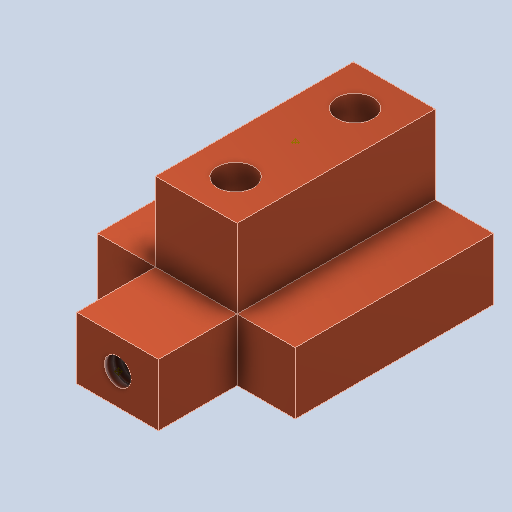
# Autodesk Inventor part: copper_top_ledgereod
Saved by Autodesk Inventor 2024.2 (Build 282272000, 272)
## iProperties
Created: 2023-03-13
Part Number: copper_top_ledgereod
Material: Copper
Document SubType Name: Modeling
Designer: warke
Density: 8.94 g/cm^3
Appearance: Copper - Satin
Author: warke
Autodesk Inventor part; units mm, degrees
ref_plane "YZ Plane" through (0, 0, 0) normal (1, 0, 0) x (0, 1, 0)
ref_plane "XZ Plane" through (0, 0, 0) normal (0, 1, 0) x (-1, 0, 0)
ref_plane "XY Plane" through (0, 0, 0) normal (0, 0, 1) x (1, 0, 0)
sketch "Sketch1" plane through (0, 0, 0) normal (0, 1, 0) x (-1, 0, 0)
  point P0 (0, 0)
sketch "Sketch2" plane through (0, 0, 0) normal (0, 1, 0) x (-1, 0, 0)
  line L0 (3.3, 8) -> (-3.3, 8)
  line L1 (-3.3, 8) -> (-3.3, -8)
  line L2 (-3.3, -8) -> (3.3, -8)
  line L3 (3.3, -8) -> (3.3, 8)
  line L4 (3.3, 8) -> (-3.3, -8) construction
  line L5 (-3.3, 8) -> (3.3, -8) construction
  point P0 (0, 0)
  dimension "d0" = 6.6
  dimension "d1" = 16
  constraints: 12 end point, 2 midpoint, 2 parallel, 1 horizontal, 1 perpendicular
  measures "d0" distance of L2.end L1.end
  measures "d1" distance of L1.end L0.end
extrude "Extrusion1" add sketch "Sketch2" along normal blind 6.35
sketch "Sketch3" plane through (0, 0, 0) normal (0, -1, 0) x (1, 0, 0)
  line L0 (-8, -8) -> (8, -8)
  line L1 (8, -8) -> (8, 8)
  line L2 (8, 8) -> (-8, 8)
  line L3 (-8, 8) -> (-8, -8)
  line L4 (-8, -8) -> (8, 8) construction
  line L5 (8, -8) -> (-8, 8) construction
  point P0 (0, 0)
  dimension "d13" = 16
  dimension "d14" = 16
  constraints: 12 end point, 2 midpoint, 2 parallel, 1 horizontal, 1 perpendicular
  measures "d13" distance of L2.end L1.end
  measures "d14" distance of L1.end L0.end
move or copy body "Move1" bodies to move or copy 1 copy no translate (0, 6.35, 0)
extrude "Extrusion2" add sketch "Sketch3" against normal up to surface (6.35 mm away)
chamfer "Chamfer1" [suppressed]
chamfer "Chamfer2" [suppressed]
sketch "Sketch4" plane through (-3.3, 12.7, -8) normal (0, 1, 0) x (1, 0, 0)
  line L0 (4.4354, -16) -> (2.1646, -16) projected
  line L1 (-4.7, 0) -> (11.3, 0) projected
  point P0 (3.3, -8)
  point P1 (3.3, -3.175)
  point P2 (3.3, -12.825)
fillet "Fillet1" [suppressed]
sketch "Sketch5" plane through (-3.3, 12.7, 8) normal (0, 0, 1) x (1, 0, 0)
  circle A0 centre (3.3, -9.5232) radius 2.9337
  point P0 (3.3, -12.7)
  constraints: 1 centre point, 1 coincident
extrude "Extrusion3" [suppressed]
hole "Hole3" [suppressed]
chamfer "Chamfer3" [suppressed]
sketch "Sketch6" plane through (-3.3, 12.7, -8) normal (-1, 0, 0) x (0, 0, 1)
  line L0 (0, 0) -> (16, 0) projected
  circle A0 centre (8, -2.27) radius 1.27
  point P0 (8, -12.7)
  dimension "d62" = 2.54
  constraints: 1 centre point
  measures "d62" diameter of A0
extrude "Extrusion4" cut sketch "Sketch6" against normal blind 3.3
sketch "Sketch7" plane through (-3.3, 12.7, 8) normal (0, 0, 1) x (1, 0, 0)
  line L0 (0, -6.35) -> (0, 0) projected
  line L1 (11.3, -12.7) -> (-4.7, -12.7) projected
  line L2 (0, -6.35) -> (6.6, -6.35)
  line L3 (6.6, -6.35) -> (6.6, -12.7)
  line L4 (6.6, -12.7) -> (0, -12.7)
  line L5 (0, -12.7) -> (0, -6.35)
  point P0 (3.3, -12.7)
  dimension "d65" = 6.6
  constraints: 8 end point, 2 parallel, 1 horizontal, 1 perpendicular, 1 point on line
  measures "d65" distance of L3.end L4.end
extrude "Extrusion5" add sketch "Sketch7" along normal blind 6.35
sketch "Sketch8" plane through (0, 0, 0) normal (0, -1, 0) x (1, 0, 0)
  line L0 (-8, 8) -> (-8, -8) projected
  line L1 (-8, -8) -> (-8, 8)
  line L2 (-3.3, 8) -> (-8, 8) projected
  line L3 (-8, 8) -> (-3.3, 8)
  line L4 (-3.3, 8) -> (-3.3, 14.35) projected
  line L5 (-3.3, 8) -> (-3.3, 14.35)
  line L6 (3.3, 14.35) -> (-3.3, 14.35) projected
  line L7 (-3.3, 14.35) -> (3.3, 14.35)
  line L8 (8, 8) -> (3.3, 8) projected
  line L9 (3.3, 14.35) -> (3.3, 8)
  line L10 (3.3, 8) -> (8, 8)
  line L11 (-8, -8) -> (8, -8) projected
  line L12 (8, 8) -> (8, -8)
  line L13 (8, -8) -> (-8, -8)
  point P0 (0, 0)
  constraints: 16 end point, 4 collinear, 3 perpendicular, 1 vertical
hole "Hole4" at (0, 12.7, 4.825) at (0, 12.7, -4.825) direction (0, -1, 0) diameter 2.946 end through all clearance for "Flat Head Machine Screw (82)" size "#4" standard "Ansi Unified Screw Threads"
extrude "Extrusion6" cut sketch "Sketch8" against normal blind 1.35
hole "Hole6" at (0, 3.85, 14.35) direction (0, 0, -1) diameter 2.1565 depth 6.35 thread size "4-40 UNC" class "2B" standard "ANSI Unified Screw Threads"
sketch "Sketch9" plane through (0, 1.35, 0) normal (0, -1, 0) x (1, 0, 0)
  point P0 (0, 0)
  point P1 (0, 0)
  constraints: 1 coincident
body "Solid1"
